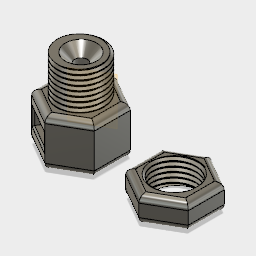
FilamentCleaner (Autodesk Fusion 360 design; units mm, degrees)
Autodesk Fusion 360 part; units mm, degrees
sketch "Sketch1" plane through (0, 0, 0) normal (0, 1, 0) x (1, 0, 0)
  line L0 (10, 5.7735) -> (0, 11.547)
  line L1 (0, 11.547) -> (-10, 5.7735)
  line L2 (-10, 5.7735) -> (-10, -5.7735)
  line L3 (-10, -5.7735) -> (0, -11.547)
  line L4 (0, -11.547) -> (10, -5.7735)
  line L5 (10, -5.7735) -> (10, 5.7735)
extrude "Extrude1" add sketch "Sketch1" along normal blind 15 makes body 1
sketch "Sketch2" plane through (0, 15, 0) normal (0, 1, 0) x (-1, 0, 0)
  line L0 (-10, 5.7735) -> (-10, -5.7735)
  line L1 (-10, -5.7735) -> (0, -11.547)
  line L2 (0, -11.547) -> (10, -5.7735)
  line L3 (10, -5.7735) -> (10, 5.7735)
  line L4 (10, 5.7735) -> (0, 11.547)
  line L5 (0, 11.547) -> (-10, 5.7735)
  circle A0 centre (0, 0) radius 7.5
  dimension "d3" = 15
  constraint coincident A0.centre origin
  measures "d3" diameter of A0
extrude "Extrude2" add sketch "Sketch2" along normal blind 12 contours A0 bodies 1
sketch "Sketch3" plane through (-5, 0, -8.6603) normal (-0.5, 0, -0.866025) x (-0.866025, 0, 0.5)
  line L0 (-5.7735, 0) -> (5.7735, 0)
  line L1 (5.7735, 0) -> (5.7735, 15)
  line L2 (5.7735, 15) -> (-5.7735, 15)
  line L3 (-5.7735, 15) -> (-5.7735, 0)
sketch "Sketch4" plane through (0, 27, 0) normal (0, 1, 0) x (-1, 0, 0)
  circle A0 centre (0, 0) radius 7.5
  circle A1 centre (0, 0) radius 2
  dimension "d6" = 4
  constraint coincident A0.centre A1.centre
  measures "d6" diameter of A1
extrude "Extrude3" cut sketch "Sketch4" against normal blind 30 contours A1 bodies 1
sketch "Sketch5" plane through (-5, 0, 8.6603) normal (-0.5, 0, 0.866025) x (0.866025, 0, 0.5)
  line L0 (-5.7735, 0) -> (5.7735, 0)
  line L1 (5.7735, 0) -> (5.7735, 15)
  line L2 (5.7735, 15) -> (-5.7735, 15)
  line L3 (-5.7735, 15) -> (-5.7735, 0)
  line L4 (-5, 10) -> (5, 10)
  line L5 (5, 10) -> (5, 5)
  line L6 (5, 5) -> (-5, 5)
  line L7 (-5, 5) -> (-5, 10)
  constraint horizontal L4
  constraint vertical L5
  constraint horizontal L6
  constraint vertical L7
extrude "Extrude4" cut sketch "Sketch5" against normal blind 15 contours L4 L5 L6 L7 bodies 1
thread "Thread1" "ISO Metric profile 15.0 M15x1.5 6g" major diameter 14.85 minor diameter 13.1369 pitch 1.5 angle 60 modelled right hand crest width 0.1875 on face at (-7.4907, 23, -0.3738) crest through (-7.425, 14.9062, 0) on bodies 1
fillet "Fillet1" radius 2 12 edges at (10, 15, 0) (5, 15, -8.6603) (-5, 15, -8.6603) (-10, 15, 0) (-5, 15, 8.6603) (5, 15, 8.6603) (-5, 0, 8.6603) (5, 0, 8.6603) (10, 0, 0) (5, 0, -8.6603) (-5, 0, -8.6603) (-10, 0, 0) on bodies 1
chamfer "Chamfer1" distance 0.5 angle 45 4 edges at (-5, 10, 8.6603) (-0.6699, 7.5, 11.1603) (-5, 5, 8.6603) (-9.3301, 7.5, 6.1603) on bodies 1
chamfer "Chamfer2" distance 5 angle 45 1 edges at (1.8647, 0, -0.7232) on bodies 1
chamfer "Chamfer3" distance 3 angle 45 1 edges at (1.8647, 27, 0.7232) on bodies 1
sketch "Sketch6" plane through (0, 0, 0) normal (0, 1, 0) x (1, 0, 0)
  line L0 (40, 5.7735) -> (30, 11.547)
  line L1 (30, 11.547) -> (20, 5.7735)
  line L2 (20, 5.7735) -> (20, -5.7735)
  line L3 (20, -5.7735) -> (30, -11.547)
  line L4 (30, -11.547) -> (40, -5.7735)
  line L5 (40, -5.7735) -> (40, 5.7735)
extrude "Extrude5" add sketch "Sketch6" along normal blind 8 separate body makes body 2
sketch "Sketch7" plane through (0, 8, 0) normal (0, 1, 0) x (-1, 0, 0)
  line L0 (-40, 5.7735) -> (-40, -5.7735)
  line L1 (-40, -5.7735) -> (-30, -11.547)
  line L2 (-30, -11.547) -> (-20, -5.7735)
  line L3 (-20, -5.7735) -> (-20, 5.7735)
  line L4 (-20, 5.7735) -> (-30, 11.547)
  line L5 (-30, 11.547) -> (-40, 5.7735)
  circle A0 centre (-30, 0) radius 7.5
  dimension "d17" = 15
  measures "d17" diameter of A0
extrude "Extrude6" cut sketch "Sketch7" against normal blind 8 contours A0 bodies 2
thread "Thread2" "ISO Metric profile 15.0 M15x1.5 6H" major diameter 15.2033 minor diameter 13.5262 pitch 1.5 angle 60 modelled right hand crest width 0.1875 on face at (22.5373, 2.6667, -0.7468) crest through (23.2369, 8.8438, 0) on bodies 2
fillet "Fillet2" radius 2 12 edges at (25, 8, 8.6603) (35, 8, 8.6603) (40, 8, 0) (35, 8, -8.6603) (25, 8, -8.6603) (20, 8, 0) (25, 0, 8.6603) (35, 0, 8.6603) (40, 0, 0) (35, 0, -8.6603) (25, 0, -8.6603) (20, 0, 0) on bodies 2
